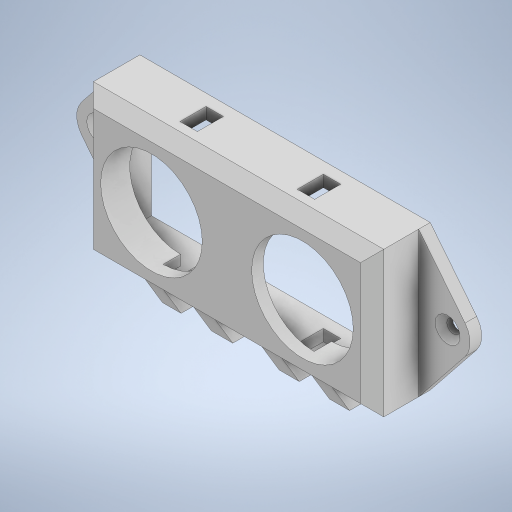
# Autodesk Inventor part: UltrasonicSensorMountTest
Saved by Autodesk Inventor 2024 (Build 280153000, 153)
## iProperties
Created: 2024-04-02
Part Number: UltrasonicSensorMountTest
Material: Generic
Document SubType Name: Modeling
Designer: ringl
Density: 1 g/cm^3
Appearance: Default
Author: ringl
Autodesk Inventor part; units mm, degrees
ref_plane "YZ Plane" through (0, 0, 0) normal (1, 0, 0) x (0, 1, 0)
ref_plane "XZ Plane" through (0, 0, 0) normal (0, 1, 0) x (-1, 0, 0)
ref_plane "XY Plane" through (0, 0, 0) normal (0, 0, 1) x (1, 0, 0)
sketch "Sketch1" plane through (0, 0, 0) normal (0, 0, 1) x (1, 0, 0)
  circle A0 centre (0, 0) radius 8.75
  circle A1 centre (26, 0) radius 8.75
  line L0 (-12, 12.5) -> (38, 12.5)
  line L1 (38, 12.5) -> (38, -12.5)
  line L2 (38, -12.5) -> (-12, -12.5)
  line L3 (-12, -12.5) -> (-12, 12.5)
  dimension "d0" = 17.5
  dimension "d1" = 17.5
  dimension "d2" = 26
  dimension "d3" = 50
  dimension "d4" = 25
  dimension "d5" = 12
  dimension "d6" = 12.5
  constraints: 8 end point, 2 centre point, 2 parallel, 1 coincident, 1 horizontal, 1 horizontal alignment, 1 perpendicular
  measures "d0" diameter of A0
  measures "d1" diameter of A1
  measures "d2" distance of point (0, 0) A1.centre
  measures "d3" distance of L1.end L2.end
  measures "d4" distance of L0.end L1.end
  measures "d5" distance from line of L3 point (0, 0)
  measures "d6" distance from line of L0 point (0, 0)
extrude "Extrusion1" add sketch "Sketch1" along normal blind 2
sketch "Sketch2" plane through (0, 0, 0) normal (0, 0, -1) x (-1, 0, 0)
  line L0 (-38, 12.5) -> (12, 12.5) projected
  line L1 (12, -12.5) -> (-38, -12.5) projected
  line L2 (-38, 12.5) -> (12, 12.5)
  line L3 (12, 12.5) -> (12, -12.5)
  line L4 (-38, -12.5) -> (-38, 12.5)
  line L5 (-36, 10.5) -> (10, 10.5)
  line L6 (10, 10.5) -> (10, -10.5)
  line L7 (-36, -10.5) -> (-36, 10.5)
  line L8 (-36, -10.5) -> (10, -10.5)
  line L9 (12, -12.5) -> (-38, -12.5)
  point P0 (0, 0)
  point P1 (12, 12.5)
  dimension "d12" = 2
  dimension "d14" = 46
  dimension "d16" = 21
  dimension "d23" = 25
  dimension "d64" = 2
  constraints: 16 end point, 3 horizontal, 2 parallel, 2 perpendicular
  measures "d12" distance between parallel lines of L4 L7
  measures "d14" distance of L5.start L5.end
  measures "d16" distance of L5.end L6.end
  measures "d23" distance of L4.start L0.start
  measures "d64" distance between parallel lines of L1 L8
extrude "Extrusion2" add sketch "Sketch2" along normal blind 8
sketch "Sketch3" plane through (0, 0, 0) normal (0, 0, -1) x (-1, 0, 0)
  circle A0 centre (-26, 0) radius 8.75 projected
  arc A1 (-26, 8.75) -> (-34.75, 0) centre (-26, 0) ccw
  line L0 (-36, 10.5) -> (-36, -10.5) projected
  line L1 (-36, 10.5) -> (-26, 10.5)
  line L2 (10, 10.5) -> (-36, 10.5) projected
  line L3 (-26, 8.75) -> (-26, 10.5)
  arc A2 (-34.75, 0) -> (-26, -8.75) centre (-26, 0) ccw
  line L4 (-26, -8.75) -> (-26, -10.5)
  line L5 (-19, -10.5) -> (-36, -10.5) projected
  line L6 (-36, -10.5) -> (-26, -10.5)
  line L7 (-36, 0) -> (-36, -10.5)
  circle A3 centre (0, 0) radius 8.75 projected
  arc A4 (8.75, 0) -> (0, 8.75) centre (0, 0) ccw
  arc A5 (0, -8.75) -> (8.75, 0) centre (0, 0) ccw
  line L8 (0, -8.75) -> (0, -10.5)
  line L9 (0, -10.5) -> (10, -10.5)
  line L10 (10, -10.5) -> (10, 10.5)
  line L11 (0, 10.5) -> (0, 8.75)
  point P0 (-26, 9.625)
  point P1 (-35.375, 0)
  point P2 (-26, -9.625)
  point P3 (0, 9.625)
  constraints: 18 end point, 14 point on circle, 5 perpendicular, 4 centre point, 4 midpoint, 4 point on line, 3 concentric, 3 vertical alignment, 2 vertical, 1 collinear
extrude "Extrusion3" add sketch "Sketch3" along normal blind 3 contours A0 L4 L5 L0 L1 L3 | L10 L9 L8 A3 L11 L2
chamfer "Chamfer2" distance 2 angle 45 4 edges at (13, 12.5, 2) (13, -12.5, 2) (38, 0, 2) (-12, 0, 2)
sketch "Sketch5" plane through (19, -12.5, -8) normal (0, -1, 0) x (1, 0, 0)
  line L0 (5.6, 2) -> (2.6, 2)
  line L1 (2.6, 2) -> (2.6, 6.5)
  line L2 (2.6, 6.5) -> (5.6, 6.5)
  line L3 (5.6, 6.5) -> (5.6, 2)
  line L4 (-14.6, 2) -> (-17.6, 2)
  line L5 (-17.6, 2) -> (-17.6, 6.5)
  line L6 (-17.6, 6.5) -> (-14.6, 6.5)
  line L7 (-14.6, 6.5) -> (-14.6, 2)
  line L8 (19, 0) -> (19, 10) projected
  line L9 (-31, 8) -> (19, 8) projected
  line L10 (19, 0) -> (-31, 0) projected
  line L11 (-31, 8) -> (19, 8) projected
  point P0 (-19, 8)
  point P1 (0, 8)
  point P2 (0, 0)
  point P3 (-12, 8)
  dimension "d29" = 3
  dimension "d31" = 3
  dimension "d33" = 17.2
  dimension "d34" = 13.4
  dimension "d35" = 1.5
  dimension "d38" = 2
  dimension "d39" = 1.5
  constraints: 16 end point, 4 parallel, 2 horizontal, 2 perpendicular, 1 point on line
  measures "d29" distance of L1.end L2.end
  measures "d31" distance of L5.end L6.end
  measures "d33" distance between parallel lines of L7 L1
  measures "d34" distance between parallel lines of L8 L3
  measures "d35" distance between parallel lines of L2 L9
  measures "d38" distance between parallel lines of L10 L0
  measures "d39" distance between parallel lines of L11 L6
extrude "Extrusion4" cut sketch "Sketch5" against normal through all
sketch "Sketch6" plane through (0, 0, -8) normal (0, 0, -1) x (-1, 0, 0)
  line L0 (12, 12.5) -> (-38, 12.5) projected
  line L1 (-38, 12.5) -> (-48, 0)
  line L2 (-36, -10.5) -> (-38, -12.5) projected
  line L3 (-48, 0) -> (-38, -12.5)
  line L4 (-38, 12.5) -> (-38, -12.5) projected
  circle A0 centre (-43, 0) radius 1.15
  line L5 (12, -12.5) -> (12, 12.5) projected
  line L6 (12, 12.5) -> (22, 0)
  line L7 (22, 0) -> (12, -12.5)
  circle A1 centre (17, 0) radius 1.15
  point P0 (0, 0)
  point P1 (-38, 0)
  dimension "d40" = 10
  dimension "d41" = 2.3
  dimension "d42" = 5
  dimension "d47" = 10
  dimension "d48" = 2.3
  dimension "d49" = 5
  constraints: 8 end point, 4 horizontal alignment, 2 centre point, 1 midpoint
  measures "d40" distance from line of L4 L1.end
  measures "d41" diameter of A0
  measures "d42" distance of point (-38, 0) A0.centre
  measures "d47" distance from line of L5 L6.end
  measures "d48" diameter of A1
  measures "d49" distance from line of L5 A1.centre
extrude "Extrusion5" add sketch "Sketch6" against normal blind 2
fillet "Fillet1" radius 4 2 edges at (48, 0, -7) (-22, 0, -7)
chamfer "Chamfer3" distance 1 angle 45 2 edges at (44.15, 0, -6) (-15.85, 0, -6)
ref_plane "Work Plane2" through (-3.1, -12.5, 0) normal (-1, 0, 0) x (0, 0, 1)
sketch "Sketch8" plane through (-3.1, -12.5, 0) normal (-1, 0, 0) x (0, 0, 1)
  line L0 (0, 0) -> (-8, 0) projected
  line L1 (0, 0) -> (-3, -5)
  line L2 (-3, -5) -> (-8, -5)
  line L3 (-8, -5) -> (-8, 0)
  line L4 (-8, 0) -> (0, 0)
  point P0 (0, 12.5)
  dimension "d56" = 5
  dimension "d57" = 5
  constraints: 8 end point, 1 collinear, 1 parallel, 1 perpendicular
  measures "d56" distance between parallel lines of L0 L2
  measures "d57" distance of L1.end L2.end
extrude "Extrusion6" add sketch "Sketch8" against normal blind 12.1
ref_plane "Work Plane4" through (29.1, -12.5, 0) normal (1, 0, 0) x (0, 0, -1)
sketch "Sketch10" plane through (29.1, -12.5, 0) normal (1, 0, 0) x (0, 0, -1)
  line L0 (8, 0) -> (0, 0) projected
  line L1 (3, -5) -> (0, 0) projected
  line L2 (0, 0) -> (3, -5)
  line L3 (8, 0) -> (8, -5) projected
  line L4 (3, -5) -> (8, -5)
  line L5 (8, -5) -> (8, 0)
  line L6 (8, 0) -> (8, -5)
  line L7 (8, 0) -> (0, 0)
  point P0 (0, 12.5)
  constraints: 10 end point, 3 perpendicular, 2 collinear
extrude "Extrusion7" add sketch "Sketch10" against normal blind 12.1
sketch "Sketch13" plane through (29.1, -17.5, -8) normal (0, -1, 0) x (1, 0, 0)
  line L0 (6.9, 0) -> (-39.1, 0) projected
  line L1 (-29.1, 8) -> (-3.1, 8) projected
  line L2 (-3.45, 0) -> (-8.65, 0)
  line L3 (-8.65, 0) -> (-8.65, 8)
  line L4 (-8.65, 8) -> (-3.45, 8)
  line L5 (-3.45, 8) -> (-3.45, 0)
  line L6 (-23.8, 0) -> (-29, 0)
  line L7 (-29, 0) -> (-29, 8)
  line L8 (-29, 8) -> (-23.8, 8)
  line L9 (-23.8, 8) -> (-23.8, 0)
  line L10 (0, 5) -> (0, 0) projected
  line L11 (-20.1, 5) -> (-20.1, 0) projected
  point P0 (-23.8, 0)
  point P1 (-23.8, 8)
  point P2 (-29, 0)
  point P3 (-8.65, 0)
  dimension "d65" = 5.2
  dimension "d66" = 3.45
  dimension "d67" = 3.7
  dimension "d68" = 5.2
  constraints: 16 end point, 4 parallel, 4 point on line, 2 horizontal, 2 perpendicular
  measures "d65" distance between parallel lines of L5 L3
  measures "d66" distance between parallel lines of L10 L5
  measures "d67" distance between parallel lines of L9 L11
  measures "d68" distance between parallel lines of L9 L7
extrude "Extrusion8" cut sketch "Sketch13" against normal blind 5 contours L0 L3 L1 L5 | L0 L7 L1 L9
body "Solid1"
